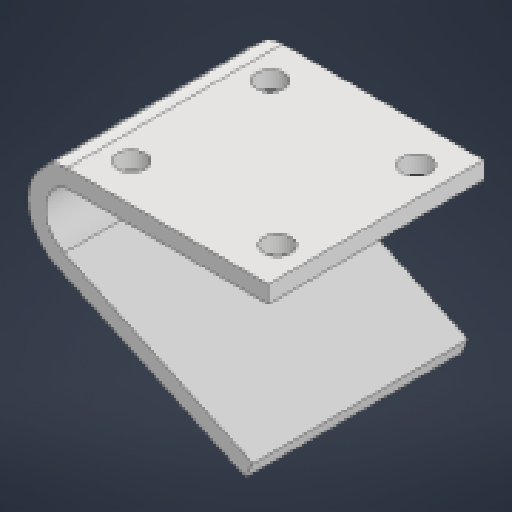
# Autodesk Inventor part: helmet_holder
Saved by Autodesk Inventor 2024 (Build 280153000, 153)
## iProperties
Created: 2026-08-20
Part Number: helmet_holder
Material: Generic
Document SubType Name: Modeling
Designer: schar
Density: 1 g/cm^3
Appearance: Default
Author: schar
Autodesk Inventor part; units mm, degrees
ref_plane "YZ Plane" through (0, 0, 0) normal (1, 0, 0) x (0, 1, 0)
ref_plane "XZ Plane" through (0, 0, 0) normal (0, 1, 0) x (-1, 0, 0)
sketch "Sketch1" plane through (0, 0, 0) normal (0, 0, 1) x (1, 0, 0)
  line L0 (0, 0) -> (27.1892, -12.6785) projected
  line L1 (-1.0565, -2.2658) -> (26.1327, -14.9443) projected
  line L2 (-1.8478, -3.9627) -> (0.8452, 1.8126) projected
  line L3 (27.1892, -12.6785) -> (26.1327, -14.9443) projected
  line L4 (29.393, 8.2928) -> (0.4528, 8.2928)
  arc A0 (-0.6947, 7.9309) -> (0, 0) centre (1.9427, 4.166) ccw
  arc A1 (0.4528, 8.2928) -> (-0.6947, 7.9309) centre (0.4528, 6.2928) ccw
  arc A2 (-2.129, 9.9785) -> (-1.0565, -2.2658) centre (1.9427, 4.166) ccw
  arc A3 (0.4528, 10.7928) -> (-2.129, 9.9785) centre (0.4528, 6.2928) ccw
  line L5 (0.4528, 10.7928) -> (29.393, 10.7928)
  line L6 (29.393, 8.2928) -> (29.393, 10.7928)
  point P0 (-0.082, 8.2928)
  dimension "d2" = 2
  constraints: 9 point on circle, 6 end point, 4 centre point, 3 tangent, 1 horizontal, 1 perpendicular, 1 point on line, 2 other
  measures "d2" radius of A1
ref_plane "Work Plane1" through (-1.0565, -14.9443, 31) normal (0, 0, -1) x (0, 1, 0)
extrude "Extrusion1" add sketch "Sketch1" along normal up to surface (31 mm away)
sketch "Sketch2" plane through (0.4528, 10.7928, 0) normal (0, 1, 0) x (1, 0, 0)
  line L0 (28.9401, 0) -> (28.9401, -31) projected
  line L1 (0, 0) -> (0, -31) projected
  line L2 (28.9401, 0) -> (0, 0)
  line L3 (0, 0) -> (0, -15.5)
  line L4 (0, -15.5) -> (28.9401, -15.5)
  line L5 (28.9401, -15.5) -> (28.9401, 0)
  line L6 (24.7213, -15.5) -> (28.7213, -15.5)
  line L7 (24.7213, -15.5) -> (24.7213, -25.5)
  line L8 (24.7213, -25.5) -> (3.7213, -25.5)
  line L9 (3.7213, -25.5) -> (3.7213, -5.5)
  line L10 (3.7213, -5.5) -> (24.7213, -5.5)
  line L11 (24.7213, -5.5) -> (24.7213, -25.5)
  circle A0 centre (24.7213, -5.5) radius 2
  circle A1 centre (24.7213, -25.5) radius 2
  circle A2 centre (3.7213, -25.5) radius 2
  circle A3 centre (3.7213, -5.5) radius 2
  point P0 (-0.4528, 0)
  dimension "d5" = 4
  dimension "d6" = 10
  dimension "d7" = 21
  dimension "d8" = 20
  dimension "d9" = 4
  dimension "d10" = 4
  dimension "d11" = 4
  dimension "d12" = 4
  constraints: 20 end point, 4 centre point, 4 coincident, 4 parallel, 2 horizontal, 2 perpendicular, 2 point on line, 1 midpoint, 1 vertical
  measures "d5" distance of L6.start L6.end
  measures "d6" distance of L6.start L7.end
  measures "d7" distance of L9.end L10.end
  measures "d8" distance of L8.end L9.end
  measures "d9" diameter of A0
  measures "d10" diameter of A1
  measures "d11" diameter of A2
  measures "d12" diameter of A3
extrude "Extrusion2" cut sketch "Sketch2" against normal up to surface (2.5 mm away) contours A1 L8 L7 | L7 L8 A1 | A0 L10 L11 | L11 L10 A0 | A2 L8 L9 | L9 L8 A2 | A3 L10 L9 | L9 L10 A3
body "Solid1"
